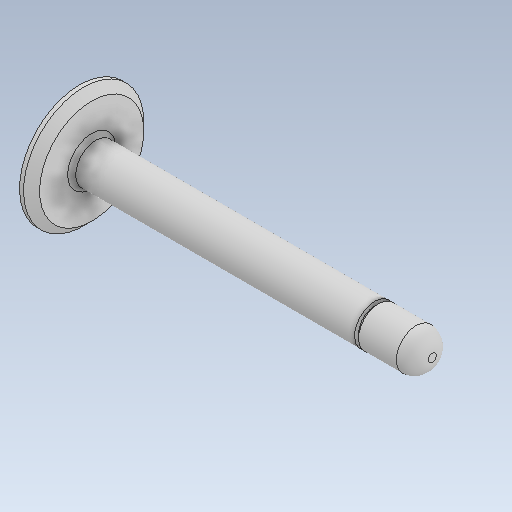
# Autodesk Inventor part: Peça7
Saved by Autodesk Inventor 2021 (Build 250183000, 183)
## iProperties
Category: 41
Created: 2021-07-27
Part Number: Peça7
Material: Genérico
Document SubType Name: Modeling
Designer: Giovanni
Density: 1 g/cm^3
Appearance: Padrão
User Status: 1:1
Author: Giovanni
Keywords: 13
Autodesk Inventor part; units mm, degrees
ref_plane "YZ Plane" through (0, 0, 0) normal (1, 0, 0) x (0, 1, 0)
ref_plane "XZ Plane" through (0, 0, 0) normal (0, 1, 0) x (-1, 0, 0)
ref_plane "XY Plane" through (0, 0, 0) normal (0, 0, 1) x (1, 0, 0)
sketch "Esboço1" plane through (0, 0, 0) normal (0, 0, 1) x (1, 0, 0)
  line L0 (0, 0) -> (88, 0)
  line L1 (88, 0) -> (88, 5)
  line L2 (88, 5) -> (3, 5)
  line L3 (3, 5) -> (3, 15)
  line L4 (3, 15) -> (0, 15)
  line L5 (0, 15) -> (0, 0)
  dimension "d0" = 88
  dimension "d1" = 5
  dimension "d2" = 3
  dimension "d3" = 15
  constraints: 12 end point, 5 perpendicular, 1 horizontal
  measures "d0" distance of L0.start L0.end
  measures "d1" distance between parallel lines of L2 L0
  measures "d2" distance of L3.end L4.end
  measures "d3" distance of L0.start L4.end
revolve "Revolução1" add sketch "Esboço1" angle 360 about axis through (0, 0, 0) along (1, 0, 0)
chamfer "Chanfro1" distance 2 angle 45 1 edges at (3, -15, 0)
fillet "Arredondamento1" radius 4 1 edges at (88, -5, 0)
fillet "Arredondamento2" radius 1 1 edges at (3, -5, 0)
sketch "Esboço2" plane through (0, 0, 0) normal (0, 0, 1) x (1, 0, 0)
  line L0 (4, 5) -> (84, 5) projected
  line L1 (73.6, 5) -> (74.6, 5)
  line L2 (74.6, 5) -> (74.6, 4)
  line L3 (74.6, 4) -> (73.6, 4)
  line L4 (73.6, 4) -> (73.6, 5)
  line L5 (-17.6, 0) -> (105.6, 0) projected
  point P0 (0, 0)
  dimension "d10" = 1
  dimension "d11" = 4
  dimension "d12" = 73.6
  constraints: 8 end point, 2 parallel, 1 horizontal, 1 perpendicular, 1 point on line
  measures "d10" distance between parallel lines of L2 L4
  measures "d11" distance from line of point (0, 0) L3
  measures "d12" distance from line of point (0, 0) L4
revolve "Revolução2" cut sketch "Esboço2" angle 360 about axis through (-10, 0, 0) along (1, 0, 0)
